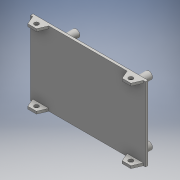
# Autodesk Inventor part: Pi Holder
Saved by Autodesk Inventor 2016 (Build 200138000, 138)
## iProperties
Created: 2018-01-17
Part Number: Pi Holder
Material: Generic
Document SubType Name: Modeling
Designer: trevo
Density: 1 g/cm^3
Appearance: Default
Author: trevo
Autodesk Inventor part; units mm, degrees
ref_plane "YZ Plane" through (0, 0, 0) normal (1, 0, 0) x (0, 1, 0)
ref_plane "XZ Plane" through (0, 0, 0) normal (0, 1, 0) x (-1, 0, 0)
ref_plane "XY Plane" through (0, 0, 0) normal (0, 0, 1) x (1, 0, 0)
sketch "Sketch1" plane through (0, 0, 0) normal (0, 1, 0) x (-1, 0, 0)
  line L0 (0, 0) -> (92.5, 0)
  line L1 (92.5, 0) -> (92.5, -59.5)
  line L2 (92.5, -59.5) -> (0, -59.5)
  line L3 (0, -59.5) -> (0, 0)
  dimension "d0" = 92.5
  dimension "d1" = 59.5
  constraints: 8 end point, 2 parallel, 1 horizontal, 1 perpendicular
  measures "d0" distance of L0.start L0.end
  measures "d1" distance of L2.end L0.start
extrude "Extrusion1" add sketch "Sketch1" along normal blind 2
sketch "Sketch2" plane through (0, 0, -59.5) normal (0, 0, -1) x (-1, 0, 0)
  line L0 (0, 0) -> (92.5, 0) projected
  line L1 (46.25, 0) -> (46.25, 2) construction
  line L2 (92.5, 2) -> (0, 2) projected
  line L3 (14.75, 0) -> (1.75, 0)
  line L4 (4.75, -7) -> (11.75, -7)
  line L5 (1.75, 0) -> (4.75, -7)
  line L6 (14.75, 0) -> (11.75, -7)
  circle A0 centre (8.25, -3.5) radius 1.75
  line L7 (87.75, -7) -> (80.75, -7)
  line L8 (90.75, 0) -> (87.75, -7)
  line L9 (77.75, 0) -> (80.75, -7)
  circle A1 centre (84.25, -3.5) radius 1.75
  line L10 (90.75, 0) -> (77.75, 0)
  dimension "d4" = 13
  dimension "d5" = 7
  dimension "d6" = 1.75
  dimension "d7" = 7
  dimension "d8" = 3
  dimension "d9" = 3.5
  dimension "d10" = 6.5
  dimension "d11" = 3.5
  constraints: 18 end point, 5 symmetric about line, 2 centre point, 2 midpoint, 1 collinear, 1 horizontal, 1 parallel, 1 point on line, 1 other
  measures "d4" distance of L3.start L3.end
  measures "d5" distance between parallel lines of L4 L0
  measures "d6" distance of L0.start L3.end
  measures "d7" distance of L4.start L4.end
  measures "d8" horizontal distance of L4.end L3.start
  measures "d9" diameter of A0
  measures "d10" horizontal distance of L3.end A0.centre
  measures "d11" distance from line of L0 A0.centre
extrude "Extrusion2" add sketch "Sketch2" against normal up to surface (59.5 mm away)
sketch "Sketch3" plane through (0, 0, 0) normal (0, -1, 0) x (1, 0, 0)
  line L0 (-92.5, -57.5) -> (0, -57.5)
  line L1 (0, -57.5) -> (0, -2)
  line L2 (0, -2) -> (-92.5, -2)
  line L3 (-92.5, -2) -> (-92.5, -57.5)
  line L4 (-77.75, -59.5) -> (-14.75, -59.5) projected
  line L5 (-92.5, -59.5) -> (-92.5, 0) projected
  line L6 (-14.75, 0) -> (-77.75, 0) projected
  line L7 (0, 0) -> (0, -59.5) projected
  dimension "d14" = 2
  dimension "d16" = 0
  dimension "d17" = 2
  dimension "d18" = 0
  constraints: 8 end point, 2 parallel, 1 horizontal, 1 perpendicular
  measures "d14" distance between parallel lines of L4 L0
  measures "d16" distance between parallel lines of L5 L3
  measures "d17" distance between parallel lines of L6 L2
  measures "d18" distance between parallel lines of L7 L1
extrude "Extrusion3" cut sketch "Sketch3" along normal through all
sketch "Sketch4" plane through (0, 2, 0) normal (0, 1, 0) x (1, 0, 0)
  line L0 (-89, 0.8) -> (-4, 0.8) construction
  line L1 (-4, 0.8) -> (-4, 56.8) construction
  line L2 (-4, 56.8) -> (-89, 56.8) construction
  line L3 (-89, 56.8) -> (-89, 0.8) construction
  line L4 (0, 0) -> (0, 59.5) projected
  line L5 (-92.5, 0) -> (0, 0) projected
  circle A0 centre (-7.5, 4.3) radius 3
  circle A1 centre (-7.5, 53.3) radius 3
  circle A2 centre (-66, 4.3) radius 3
  circle A3 centre (-66, 53.3) radius 3
  circle A4 centre (-66, 4.3) radius 1.75
  circle A5 centre (-66, 53.3) radius 1.75
  circle A6 centre (-7.5, 53.3) radius 1.75
  circle A7 centre (-7.5, 4.3) radius 1.75
  dimension "d21" = 85
  dimension "d22" = 56
  dimension "d23" = 4
  dimension "d24" = 0.8
  dimension "d25" = 6
  dimension "d26" = 6
  dimension "d27" = 6
  dimension "d28" = 6
  dimension "d29" = 3.5
  dimension "d30" = 3.5
  dimension "d31" = 3.5
  dimension "d32" = 3.5
  dimension "d33" = 3.5
  dimension "d34" = 3.5
  dimension "d35" = 58.5
  dimension "d36" = 58.5
  dimension "d37" = 3.5
  dimension "d38" = 3.5
  dimension "d39" = 3.5
  dimension "d40" = 3.5
  constraints: 8 centre point, 8 end point, 4 coincident, 2 parallel, 1 horizontal, 1 perpendicular
  measures "d21" distance of L0.start L0.end
  measures "d22" distance of L0.end L1.end
  measures "d23" distance between parallel lines of L4 L1
  measures "d24" distance between parallel lines of L5 L0
  measures "d25" diameter of A3
  measures "d26" diameter of A2
  measures "d27" diameter of A0
  measures "d28" diameter of A1
  measures "d29" distance from line of L1 A1.centre
  measures "d30" distance from line of L2 A1.centre
  measures "d31" distance from line of L1 A0.centre
  measures "d32" distance from line of L0 A0.centre
  measures "d33" distance from line of L0 A2.centre
  measures "d34" distance from line of L2 A3.centre
  measures "d35" distance of A3.centre A1.centre
  measures "d36" distance of A2.centre A0.centre
  measures "d37" diameter of A4
  measures "d38" diameter of A5
  measures "d39" diameter of A6
  measures "d40" diameter of A7
extrude "Extrusion4" add sketch "Sketch4" along normal blind 8.2
body "Solid1"
